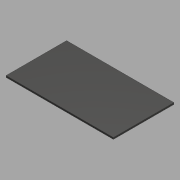
# Autodesk Inventor part: Battery Case Top
Saved by Autodesk Inventor 2017 (Build 210142000, 142)
## iProperties
Created: 2017-05-08
Part Number: Battery Case Top
Material: ABS Plastic
Document SubType Name: Modeling
Designer: zallen
Density: 1.06 g/cm^3
Appearance: Smooth - Black
Mass: 18.9655 g
Surface Area: 186.8 cm^2
Volume: 17.892 cm^3
Author: zallen
Autodesk Inventor part; units mm, degrees
ref_plane "YZ Plane" through (0, 0, 0) normal (1, 0, 0) x (0, 1, 0)
ref_plane "XZ Plane" through (0, 0, 0) normal (0, 1, 0) x (-1, 0, 0)
ref_plane "XY Plane" through (0, 0, 0) normal (0, 0, 1) x (1, 0, 0)
sketch "Sketch1" plane through (0, 0, 0) normal (0, 0, 1) x (1, 0, 0)
  line L0 (0, 0) -> (126, 0)
  line L1 (126, 0) -> (126, 71)
  line L2 (126, 71) -> (0, 71)
  line L3 (0, 71) -> (0, 0)
  dimension "d0" = 126
  dimension "d1" = 71
  constraints: 8 end point, 2 parallel, 1 horizontal, 1 perpendicular
  measures "d0" distance of L2.end L1.end
  measures "d1" distance of L1.end L0.end
extrude "Extrusion1" add sketch "Sketch1" along normal blind 2
body "Solid1"
